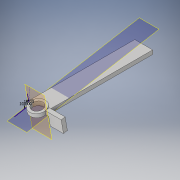
# Autodesk Inventor part: WheelIntakeMotorMount2.0
Saved by Autodesk Inventor 2017 (Build 210142000, 142)
## iProperties
Created: 2017-11-18
Part Number: WheelIntakeMotorMount2.0
Material: Generic
Document SubType Name: Modeling
Designer: User
Density: 1 g/cm^3
Appearance: Default
Author: User
Autodesk Inventor part; units mm, degrees
ref_plane "YZ Plane" through (0, 0, 0) normal (1, 0, 0) x (0, 1, 0)
ref_plane "XZ Plane" through (0, 0, 0) normal (0, 1, 0) x (-1, 0, 0)
ref_plane "XY Plane" through (0, 0, 0) normal (0, 0, 1) x (1, 0, 0)
sketch "Sketch1" plane through (0, 0, 0) normal (1, 0, 0) x (0, 1, 0)
  line L0 (0, 0) -> (21.59, 0)
  line L1 (21.59, 0) -> (21.59, -127)
  line L2 (21.59, -127) -> (0, -127)
  line L3 (0, -127) -> (0, 0)
  dimension "d0" = 21.59
  dimension "d1" = 127
  constraints: 8 end point, 2 parallel, 1 horizontal, 1 perpendicular
  measures "d0" distance of L1.end L2.end
  measures "d1" distance of L0.end L1.end
extrude "Extrusion1" add sketch "Sketch1" along normal blind 4.7625
sketch "Sketch2" plane through (0, 21.59, 0) normal (0, 1, 0) x (1, 0, 0)
  line L0 (0, 0) -> (-3.2071, -18.1884)
  line L1 (0, 0) -> (18.469, 0) construction
  line L2 (0, 0) -> (13.0579, -2.3025)
  line L3 (0, 0) -> (13.2594, 0) construction
  dimension "d4" = 100
  dimension "d24" = 10
  constraints: 8 end point, 2 equal length, 2 horizontal
  measures "d4" angle of L0 L1
  measures "d24" angle of L2 L3
ref_plane "Work Plane1" through (0, 21.59, 0) normal (-0.9848078, 0, -0.1736482) x (-0.1736482, 0, 0.9848078)
sketch "Sketch3" plane through (0, 21.59, 0) normal (-0.9848078, 0, -0.1736482) x (-0.1736482, 0, 0.9848078)
  line L0 (-0.827, 0) -> (-0.827, -21.59) projected
  line L1 (-0.827, -21.59) -> (-125.8976, -21.59) projected
  line L2 (-125.8976, -21.59) -> (-125.8976, 0) projected
  line L3 (-125.8976, 0) -> (-0.827, 0) projected
  line L4 (0, -21.59) -> (0, 0) projected
  line L5 (0, -21.59) -> (-0.827, -21.59) projected
  line L6 (-0.827, 0) -> (-0.827, -21.59) projected
  line L7 (0, 0) -> (-0.827, 0) projected
  line L8 (0, -21.59) -> (0, 0) projected
  circle A0 centre (0, -10.795) radius 9.525
  dimension "d5" = 19.05
  dimension "d6" = 21.59
  dimension "d7" = 10.795
  constraints: 1 centre point, 1 midpoint
  measures "d5" diameter of A0
  measures "d6" distance of L4.start L4.end
  measures "d7" distance from line of L7 A0.centre
extrude "Extrusion2" add sketch "Sketch3" against normal blind 4.7625 contours A0 L4 L0 | L0 A0 | A0 L4
sketch "Sketch5" plane through (4.6901, 10.795, 0.827) normal (0.9848078, 0, 0.1736482) x (0.1736482, 0, -0.9848078)
  circle A0 centre (0, 0) radius 9.525 projected
  point P0 (0, -10.795)
hole "Hole2" at (4.6901, 10.795, 0.827) direction (-0.9848078, 0, -0.1736482) diameter 12.954 end through all
ref_plane "Work Plane3" through (0, 0, 0) normal (-0.1736482, 0, 0.9848078) x (0, 1, 0)
sketch "Sketch7" plane through (0, 0, 0) normal (-0.1736482, 0, 0.9848078) x (0, 1, 0)
  ellipse E0 centre (10.795, 0) end of major axis (10.795, -54.019) minor radius 9.525 (20.284, -4.6901) -> (20.32, 0) ccw projected
  line L0 (20.32, 0) -> (1.27, 0) projected
  ellipse E1 centre (10.795, 0) end of major axis (10.795, -54.019) minor radius 9.525 (1.27, 0) -> (1.306, -4.6901) ccw projected
  ellipse E2 centre (10.795, -4.836) end of major axis (1.27, -4.836) minor radius 1.6795 (20.284, -4.6901) -> (1.306, -4.6901) ccw projected
  line L1 (1.27, -4.7625) -> (20.32, -4.7625) projected
  ellipse E3 centre (10.795, 0) end of major axis (10.795, -54.019) minor radius 9.525 (1.27, 0) -> (1.306, -4.6901) ccw projected
  line L2 (0, 0) -> (1.27, 0) projected
  line L3 (0, 0) -> (0, -4.6901) projected
  line L4 (1.306, -4.6901) -> (0, -4.6901) projected
  line L5 (1.306, -4.6901) -> (-17.744, -4.6901)
  line L6 (-17.744, -4.6901) -> (-17.744, 0)
  line L7 (-1.869, 0) -> (1.306, 0)
  line L8 (1.306, 0) -> (1.306, -4.6901)
  line L9 (-17.744, -4.6901) -> (-1.869, -4.6901)
  line L10 (-1.869, 0) -> (-1.869, 11.1849)
  line L11 (-1.869, 11.1849) -> (-17.744, 11.1849)
  line L12 (-17.744, 11.1849) -> (-17.744, -4.6901)
  dimension "d26" = 19.05
  dimension "d27" = 15.875
  dimension "d28" = 15.875
  constraints: 16 end point, 4 parallel, 2 horizontal, 2 perpendicular, 4 other
  measures "d26" distance of L6.end L7.end
  measures "d27" distance of L11.end L10.end
  measures "d28" distance of L10.end L9.end
extrude "Extrusion3" add sketch "Sketch7" against normal blind 4.7625 contours L4 L3 L2 E1 | E1 L0 L8 | L5 L6 L12 L11 L10 L7 L3
equation "\"d7\" = 0.5 * d6"
body "Solid1"
